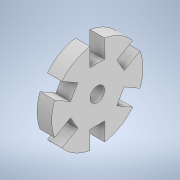
# Autodesk Inventor part: barrel_holder
Saved by Autodesk Inventor 2020.1 (Build 241239000, 239)
## iProperties
Created: 2022-03-19
Part Number: barrel_holder
Material: Типовые
Document SubType Name: Modeling
Designer: User
Density: 1 g/cm^3
Appearance: По умолчанию
Author: User
Autodesk Inventor part; units mm, degrees
ref_plane "YZ Plane" through (0, 0, 0) normal (1, 0, 0) x (0, 1, 0)
ref_plane "XZ Plane" through (0, 0, 0) normal (0, 1, 0) x (-1, 0, 0)
ref_plane "XY Plane" through (0, 0, 0) normal (0, 0, 1) x (1, 0, 0)
sketch "Эскиз1" plane through (0, 0, 0) normal (1, 0, 0) x (0, 1, 0)
  circle A0 centre (0, 0) radius 12.5
  line L0 (12.339, 2) -> (7.339, 2)
  line L1 (7.339, 2) -> (7.339, -2)
  line L2 (7.339, -2) -> (12.339, -2)
  line L3 (12.5, 0) -> (0, 0)
  line L4 (4.4374, 11.6859) -> (1.9374, 7.3557)
  line L5 (1.9374, 7.3557) -> (5.4015, 5.3557)
  line L6 (5.4015, 5.3557) -> (7.9015, 9.6859)
  line L7 (-7.9015, 9.6859) -> (-5.4015, 5.3557)
  line L8 (-5.4015, 5.3557) -> (-1.9374, 7.3557)
  line L9 (-1.9374, 7.3557) -> (-4.4374, 11.6859)
  line L10 (-12.339, -2) -> (-7.339, -2)
  line L11 (-7.339, -2) -> (-7.339, 2)
  line L12 (-7.339, 2) -> (-12.339, 2)
  line L13 (-4.4374, -11.6859) -> (-1.9374, -7.3557)
  line L14 (-1.9374, -7.3557) -> (-5.4015, -5.3557)
  line L15 (-5.4015, -5.3557) -> (-7.9015, -9.6859)
  line L16 (7.9015, -9.6859) -> (5.4015, -5.3557)
  line L17 (5.4015, -5.3557) -> (1.9374, -7.3557)
  line L18 (1.9374, -7.3557) -> (4.4374, -11.6859)
  circle A1 centre (0, 0) radius 2
  point P0 (4.4374, 11.6859)
  point P1 (-12.339, 2)
  point P2 (-12.339, -2)
  point P3 (-7.9015, -9.6859)
  point P4 (-4.4374, -11.6859)
  point P5 (4.4374, -11.6859)
  point P6 (7.9015, 9.6859)
  dimension "d2" = 360
  dimension "d4" = 5
  dimension "d5" = 25
  dimension "d8" = 4
  dimension "d9" = 4
  constraints: 38 end point, 4 coincident, 3 point on circle, 2 centre point, 2 horizontal, 1 parallel, 1 perpendicular, 48 other
  measures "d4" distance of L1.end L2.end
  measures "d5" diameter of A0
  measures "d8" diameter of A1
  measures "d9" distance of L0.end L1.end
extrude "Выдавливание1" add sketch "Эскиз1" along normal blind 4 contours L0 L1 L2 A0 L16 L17 L18 L13 L14 L15 L10 L11 L12 L7 L8 L9 L4 L5 L6
